Autodesk Fusion 360 part; units mm, degrees
note: some values were not read from the file. Chosen so that the rebuilt part matches the saved one: a direction. Set by a fixed rule: which sketch regions a step uses.
(part 5 of 5)
  spline S21 degree 5 poles (27.2031, -5.114) (27.2035, -5.1088) (27.2041, -5.0985) (27.2051, -5.0829) (27.2063, -5.0623) (27.2076, -5.0365) (27.2088, -5.0107) (27.2099, -4.985) (27.2108, -4.9594) (27.2115, -4.9338) (27.2121, -4.9082) (27.2125, -4.8827) (27.2128, -4.8573) (27.2129, -4.8319) (27.2129, -4.8066) (27.2127, -4.7813) (27.2123, -4.756) (27.2118, -4.7309) (27.2112, -4.7058) (27.2104, -4.6807) (27.2094, -4.6558) (27.2083, -4.6308) (27.207, -4.606) (27.2055, -4.5812) (27.2039, -4.5565) (27.2022, -4.5318) (27.2002, -4.5072) (27.1981, -4.4827) (27.1959, -4.4582) (27.1935, -4.4339) (27.1909, -4.4096) (27.1882, -4.3853) (27.1853, -4.3612) (27.1822, -4.3371) (27.179, -4.3131) (27.1755, -4.2892) (27.172, -4.2654) (27.1682, -4.2417) (27.1643, -4.218) (27.1602, -4.1944) (27.156, -4.171) (27.1515, -4.1476) (27.1469, -4.1243) (27.1421, -4.1011) (27.1372, -4.078) (27.132, -4.055) (27.1267, -4.0321) (27.1212, -4.0093) (27.1155, -3.9866) (27.1096, -3.964) (27.1035, -3.9415) (27.0972, -3.9192) (27.0908, -3.897) (27.0841, -3.8749) (27.0771, -3.8529) (27.07, -3.831) (27.0628, -3.8093) (27.0553, -3.7877) (27.0476, -3.7662) (27.0397, -3.7449) (27.0316, -3.7237) (27.0231, -3.7027) (27.0144, -3.682) (27.0053, -3.6614) (26.9959, -3.641) (26.9863, -3.6208) (26.9766, -3.6007) (26.9667, -3.5808) (26.9566, -3.5609) (26.9462, -3.5414) (26.935, -3.5224) (26.9254, -3.5076) (26.9178, -3.4969) (26.9124, -3.4899) (26.9097, -3.4864) knots -1 -1 -1 -1 -1 -1 -0.98571429 -0.97142857 -0.95714286 -0.94285714 -0.92857143 -0.91428571 -0.9 -0.88571429 -0.87142857 -0.85714286 -0.84285714 -0.82857143 -0.81428571 -0.8 -0.78571429 -0.77142857 -0.75714286 -0.74285714 -0.72857143 -0.71428571 -0.7 -0.68571429 -0.67142857 -0.65714286 -0.64285714 -0.62857143 -0.61428571 -0.6 -0.58571429 -0.57142857 -0.55714286 -0.54285714 -0.52857143 -0.51428571 -0.5 -0.48571429 -0.47142857 -0.45714286 -0.44285714 -0.42857143 -0.41428571 -0.4 -0.38571429 -0.37142857 -0.35714286 -0.34285714 -0.32857143 -0.31428571 -0.3 -0.28571429 -0.27142857 -0.25714286 -0.24285714 -0.22857143 -0.21428571 -0.2 -0.18571429 -0.17142857 -0.15714286 -0.14285714 -0.12857143 -0.11428571 -0.1 -0.08571429 -0.07142857 -0.05714286 -0.04285714 -0.02857143 -0.01428571 0 0 0 0 0 0
  line L21 (26.9097, -3.4864) -> (26.3684, -2.8003)
  arc A43 (26.3834, -2.6612) -> (26.3684, -2.8003) centre (26.4469, -2.7384) ccw
  arc A44 (26.3834, -2.6612) -> (27.0995, -1.945) centre (23.0613, 1.3771) ccw
  arc A45 (27.2387, -1.9301) -> (27.0995, -1.945) centre (27.1768, -2.0086) ccw
  line L22 (27.2387, -1.9301) -> (27.9248, -2.4713)
  spline S22 degree 5 poles (27.9248, -2.4713) (27.9282, -2.474) (27.9352, -2.4794) (27.946, -2.4871) (27.9607, -2.4967) (27.9798, -2.5078) (27.9993, -2.5183) (28.0191, -2.5284) (28.0391, -2.5382) (28.0592, -2.548) (28.0794, -2.5575) (28.0998, -2.5669) (28.1203, -2.576) (28.1411, -2.5847) (28.1621, -2.5932) (28.1832, -2.6013) (28.2046, -2.6092) (28.2261, -2.6169) (28.2477, -2.6244) (28.2694, -2.6317) (28.2913, -2.6388) (28.3132, -2.6457) (28.3353, -2.6524) (28.3576, -2.6589) (28.3799, -2.6651) (28.4024, -2.6712) (28.425, -2.6771) (28.4477, -2.6828) (28.4705, -2.6883) (28.4934, -2.6936) (28.5164, -2.6988) (28.5395, -2.7038) (28.5627, -2.7085) (28.5859, -2.7132) (28.6093, -2.7176) (28.6328, -2.7219) (28.6564, -2.7259) (28.68, -2.7299) (28.7038, -2.7336) (28.7276, -2.7372) (28.7515, -2.7406) (28.7755, -2.7438) (28.7996, -2.7469) (28.8237, -2.7498) (28.8479, -2.7525) (28.8722, -2.7551) (28.8966, -2.7575) (28.9211, -2.7598) (28.9456, -2.7619) (28.9702, -2.7638) (28.9948, -2.7655) (29.0196, -2.7672) (29.0444, -2.7686) (29.0692, -2.7699) (29.0941, -2.771) (29.1191, -2.772) (29.1442, -2.7728) (29.1693, -2.7735) (29.1944, -2.774) (29.2197, -2.7743) (29.2449, -2.7745) (29.2703, -2.7745) (29.2957, -2.7744) (29.3211, -2.7741) (29.3466, -2.7737) (29.3722, -2.7731) (29.3978, -2.7724) (29.4234, -2.7715) (29.4491, -2.7705) (29.4749, -2.7693) (29.5007, -2.7679) (29.5213, -2.7667) (29.5369, -2.7658) (29.5472, -2.7651) (29.5524, -2.7647) knots 0 0 0 0 0 0 0.01428571 0.02857143 0.04285714 0.05714286 0.07142857 0.08571429 0.1 0.11428571 0.12857143 0.14285714 0.15714286 0.17142857 0.18571429 0.2 0.21428571 0.22857143 0.24285714 0.25714286 0.27142857 0.28571429 0.3 0.31428571 0.32857143 0.34285714 0.35714286 0.37142857 0.38571429 0.4 0.41428571 0.42857143 0.44285714 0.45714286 0.47142857 0.48571429 0.5 0.51428571 0.52857143 0.54285714 0.55714286 0.57142857 0.58571429 0.6 0.61428571 0.62857143 0.64285714 0.65714286 0.67142857 0.68571429 0.7 0.71428571 0.72857143 0.74285714 0.75714286 0.77142857 0.78571429 0.8 0.81428571 0.82857143 0.84285714 0.85714286 0.87142857 0.88571429 0.9 0.91428571 0.92857143 0.94285714 0.95714286 0.97142857 0.98571429 1 1 1 1 1 1
  arc A46 (29.5524, -2.7647) -> (29.8938, -2.1734) centre (23.0613, 1.3771) ccw
  spline S23 degree 5 poles (29.8938, -2.1734) (29.8915, -2.1688) (29.8869, -2.1595) (29.88, -2.1455) (29.8707, -2.127) (29.8589, -2.104) (29.8471, -2.0811) (29.8351, -2.0584) (29.8231, -2.0357) (29.8109, -2.0132) (29.7986, -1.9907) (29.7863, -1.9684) (29.7738, -1.9463) (29.7612, -1.9242) (29.7485, -1.9023) (29.7357, -1.8805) (29.7228, -1.8588) (29.7098, -1.8373) (29.6966, -1.8159) (29.6834, -1.7946) (29.6701, -1.7734) (29.6566, -1.7524) (29.6431, -1.7315) (29.6295, -1.7108) (29.6157, -1.6902) (29.6018, -1.6697) (29.5879, -1.6494) (29.5738, -1.6292) (29.5596, -1.6091) (29.5454, -1.5892) (29.531, -1.5695) (29.5165, -1.5499) (29.5019, -1.5304) (29.4872, -1.5111) (29.4724, -1.4919) (29.4575, -1.4729) (29.4425, -1.4541) (29.4274, -1.4354) (29.4122, -1.4169) (29.3969, -1.3985) (29.3814, -1.3803) (29.3659, -1.3623) (29.3502, -1.3444) (29.3345, -1.3267) (29.3186, -1.3092) (29.3027, -1.2918) (29.2866, -1.2747) (29.2704, -1.2577) (29.2542, -1.2409) (29.2378, -1.2243) (29.2213, -1.2078) (29.2047, -1.1916) (29.1879, -1.1756) (29.1711, -1.1598) (29.1541, -1.1443) (29.1371, -1.1289) (29.1199, -1.1137) (29.1026, -1.0987) (29.0852, -1.084) (29.0677, -1.0694) (29.0501, -1.0551) (29.0323, -1.0412) (29.0143, -1.0276) (28.9961, -1.0144) (28.9778, -1.0014) (28.9594, -0.9887) (28.941, -0.9761) (28.9224, -0.9638) (28.9038, -0.9517) (28.885, -0.94) (28.8658, -0.9291) (28.8501, -0.9211) (28.8381, -0.9156) (28.83, -0.9122) (28.8259, -0.9106) knots -1 -1 -1 -1 -1 -1 -0.98571429 -0.97142857 -0.95714286 -0.94285714 -0.92857143 -0.91428571 -0.9 -0.88571429 -0.87142857 -0.85714286 -0.84285714 -0.82857143 -0.81428571 -0.8 -0.78571429 -0.77142857 -0.75714286 -0.74285714 -0.72857143 -0.71428571 -0.7 -0.68571429 -0.67142857 -0.65714286 -0.64285714 -0.62857143 -0.61428571 -0.6 -0.58571429 -0.57142857 -0.55714286 -0.54285714 -0.52857143 -0.51428571 -0.5 -0.48571429 -0.47142857 -0.45714286 -0.44285714 -0.42857143 -0.41428571 -0.4 -0.38571429 -0.37142857 -0.35714286 -0.34285714 -0.32857143 -0.31428571 -0.3 -0.28571429 -0.27142857 -0.25714286 -0.24285714 -0.22857143 -0.21428571 -0.2 -0.18571429 -0.17142857 -0.15714286 -0.14285714 -0.12857143 -0.11428571 -0.1 -0.08571429 -0.07142857 -0.05714286 -0.04285714 -0.02857143 -0.01428571 0 0 0 0 0 0
  line L23 (28.8259, -0.9106) -> (28.0141, -0.5871)
  arc A47 (27.9575, -0.4591) -> (28.0141, -0.5871) centre (28.0511, -0.4942) ccw
  circle A48 centre (23.0613, 1.3771) radius 1.5
  circle A49 centre (23.0613, 1.3771) radius 8.5
  dimension "d180" = 17
  constraint concentric A0 A49
extrude "Extrude3'" add sketch "Sketch6" along normal blind 3 contours A0 A1 L0 S0 A2 S1 L1 A3 A4 A5 L2 S2 A6 S3 L3 A7 A8 A9 L4 S4 A10 S5 L5 A11 A12 A13 L6 S6 A14 S7 L7 A15 A16 A17 L8 S8 A18 S9 L9 A19 A20 A21 L10 S10 A22 S11 L11 A23 A24 A25 L12 S12 A26 S13 L13 A27 A28 A29 L14 S14 A30 S15 L15 A31 A32 A33 L16 S16 A34 S17 L17 A35 A36 A37 L18 S18 A38 S19 L19 A39 A40 A41 L20 S20 A42 S21 L21 A43 A44 A45 L22 S22 A46 S23 L23 A47 | A49 sketch seen with x (1, 0, 0) y (0, 1, 0) z (0, 0, 1) at (-23.0613, -1.3771, 2.8521) bodies 8 in component "Spur Gear (12 teeth)"
move_face "OffsetFaces1" offset -2.8 1 faces at (3.9479, 0, 0) on bodies 8 in component "Spur Gear (12 teeth)"
component "Gripper (1)" placed x (0.374993, 0.927028, 0) y (-0.927028, 0.374993, 0) z (0, 0, 1) at (-28.4092, 64.7791, 0)
component "Connecting rod" placed x (-0.481274, 0.87657, 0) y (0.87657, 0.481274, 0) z (0, 0, -1) at (-11.5992, 48.8044, 6)
component "Component" placed x (1, 0, 0) y (0, 1, 0) z (0, 0, 1) at (0, 0, 0)
component "Spur Gear (24 teeth)" placed x (-0.852322, 0.523018, 0) y (-0.523018, -0.852322, 0) z (0, 0, 1) at (-13.5, 37.5997, 3)
component "Gripper" placed x (-0.375069, 0.926997, 0) y (0.926997, 0.375069, 0) z (0, 0, -1) at (31.858, 62.5794, 0)
component "Conecting Rod" placed x (0.592474, 0.80559, 0) y (-0.80559, 0.592474, 0) z (0, 0, 1) at (10.3334, 48.0473, 6)
component "Conecting Rod" placed x (0.592474, 0.80559, 0) y (0.80559, -0.592474, 0) z (0, 0, -1) at (-5.7784, 59.8968, -3)
component "Conecting Rod" placed x (0.592195, 0.805795, 0) y (0.805795, -0.592195, 0) z (0, 0, -1) at (2.4811, 39.4927, -3)
component "Connecting rod" placed x (-0.481274, 0.87657, 0) y (0.87657, 0.481274, 0) z (0, 0, -1) at (-11.5992, 48.8044, 0)
component "Connecting rod" placed x (-0.48094, 0.876753, 0) y (-0.876753, -0.48094, 0) z (0, 0, 1) at (-2.3278, 38.0254, -3)
component "Eye shape " placed x (0.80559, -0.592474, 0) y (0, 0, 1) z (-0.592474, -0.80559, 0) at (-33.5328, 5.2807, -51.0899)
component "Eye shape " placed x (0.80559, -0.592474, 0) y (0, 0, 1) z (-0.592474, -0.80559, 0) at (-15.1661, 30.254, -51.0899)
component "Eye shape " placed x (0.876753, 0.48094, 0) y (0, 0, 1) z (0.48094, -0.876753, 0) at (17.9736, -19.7767, -51.0899)
component "Eye shape " placed x (0.913767, 0.406239, 0) y (0, 0, 1) z (0.406239, -0.913767, 0) at (40.0851, -22.1989, -51.0899)
component "Eye shape " placed x (0.87657, 0.481274, 0) y (0, 0, 1) z (0.481274, -0.87657, 0) at (11.3362, 27.8093, -51.0899)
component "Eye shape " placed x (0.852322, -0.523018, 0) y (0, 0, -1) z (0.523018, 0.852322, 0) at (5.8181, 120.5566, 54.0899)
component "Eye shape " placed x (0.913767, 0.406239, 0) y (0, 0, 1) z (0.406239, -0.913767, 0) at (58.4431, 2.7807, -51.0899)
component "Eye shape " placed x (0.87657, 0.481274, 0) y (0, 0, -1) z (-0.481274, 0.87657, 0) at (-36.7353, 115.3644, 54.0899)
component "Spur Gear (12 teeth)" placed x (0.107188, -0.994239, 0) y (-0.994239, -0.107188, 0) z (0, 0, -1) at (7.5, 17.5997, 9)
component "Spur Gear (24 teeth)" placed x (0.913767, 0.406239, 0) y (0.406239, -0.913767, 0) z (0, 0, -1) at (13.5, 37.5997, 6) in component "Component"
